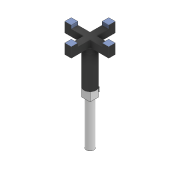
# Autodesk Inventor part: stand
Saved by Autodesk Inventor 2021 (Build 250183000, 183)
## iProperties
Created: 2021-06-25
Part Number: stand
Material: Generic
Document SubType Name: Modeling
Designer: user
Density: 1 g/cm^3
Appearance: Default
Author: user
Autodesk Inventor part; units mm, degrees
ref_plane "YZ Plane" through (0, 0, 0) normal (1, 0, 0) x (0, 1, 0)
ref_plane "XZ Plane" through (0, 0, 0) normal (0, 1, 0) x (-1, 0, 0)
ref_plane "XY Plane" through (0, 0, 0) normal (0, 0, 1) x (1, 0, 0)
sketch "Sketch1" plane through (0, 0, 0) normal (0, 1, 0) x (-1, 0, 0)
  line L0 (-127, 19.05) -> (-127, -19.05)
  line L1 (127, -19.05) -> (127, 19.05)
  line L2 (0, -127) -> (19.05, -127)
  line L3 (19.05, -127) -> (19.05, -19.05)
  line L4 (19.05, 0) -> (0, 0)
  line L5 (0, -127) -> (-19.05, -127)
  line L6 (-19.05, -127) -> (-19.05, -19.05)
  line L7 (-19.05, 0) -> (0, 0)
  line L8 (0, 0) -> (0, -127)
  line L9 (19.05, 0) -> (0, 0)
  line L10 (-19.05, 0) -> (-19.05, 127)
  line L11 (-19.05, 127) -> (19.05, 127)
  line L12 (19.05, 127) -> (19.05, 19.05)
  line L13 (-127, -19.05) -> (-19.05, -19.05)
  line L14 (19.05, -19.05) -> (127, -19.05)
  line L15 (127, 19.05) -> (19.05, 19.05)
  line L16 (-19.05, 19.05) -> (-127, 19.05)
  point P0 (127, 0)
  point P1 (-127, 0)
  point P2 (0, 19.05)
  point P3 (0, -19.05)
  dimension "d7" = 127
  dimension "d8" = 19.05
  dimension "d9" = 127
  constraints: 34 end point, 10 parallel, 5 horizontal, 5 perpendicular, 2 point on line, 1 coincident
  measures "d7" distance of L4.start L2.end
  measures "d8" distance of L4.end L7.start
  measures "d9" distance of L10.start L10.end
extrude "Extrusion1" add sketch "Sketch1" along normal blind 38.1
sketch "Sketch2" plane through (0, 38.1, 0) normal (0, 1, 0) x (1, 0, 0)
  line L0 (-19.05, -127) -> (19.05, -127) projected
  line L1 (-19.05, -127) -> (19.05, -127)
  line L2 (19.05, -127) -> (19.05, -88.9)
  line L3 (19.05, -88.9) -> (-19.05, -88.9)
  line L4 (-19.05, -88.9) -> (-19.05, -127)
  line L5 (-19.05, 127) -> (-19.05, 19.05) projected
  line L6 (19.05, 19.05) -> (19.05, 127) projected
  line L7 (-19.05, 127) -> (19.05, 127)
  line L8 (19.05, 127) -> (19.05, 88.9)
  line L9 (19.05, 88.9) -> (-19.05, 88.9)
  line L10 (-19.05, 88.9) -> (-19.05, 127)
  line L11 (-127, -19.05) -> (-19.05, -19.05) projected
  line L12 (-19.05, 19.05) -> (-127, 19.05) projected
  line L13 (-127, -19.05) -> (-88.9, -19.05)
  line L14 (-88.9, -19.05) -> (-88.9, 19.05)
  line L15 (-88.9, 19.05) -> (-127, 19.05)
  line L16 (-127, 19.05) -> (-127, -19.05)
  line L17 (127, -19.05) -> (127, 19.05) projected
  line L18 (127, 19.05) -> (19.05, 19.05) projected
  line L19 (127, -19.05) -> (88.9, -19.05)
  line L20 (88.9, -19.05) -> (88.9, 19.05)
  line L21 (88.9, 19.05) -> (127, 19.05)
  line L22 (127, 19.05) -> (127, -19.05)
  point P0 (0, 0)
  point P1 (-19.05, 88.9)
  dimension "d12" = 38.1
  dimension "d13" = 38.1
  dimension "d14" = 38.1
  dimension "d15" = 38.1
  dimension "d16" = 38.1
  constraints: 32 end point, 8 parallel, 4 horizontal, 4 perpendicular, 3 point on line
  measures "d12" distance of L3.end L2.end
  measures "d13" distance of L2.end L1.end
  measures "d14" distance of L7.end L8.end
  measures "d15" distance of L15.end L14.end
  measures "d16" distance of L20.end L21.end
extrude "Extrusion2" add sketch "Sketch2" along normal blind 19.05
sketch "Sketch3" plane through (0, 0, 0) normal (0, -1, 0) x (1, 0, 0)
  circle A0 centre (0, 0) radius 38.1
  dimension "d19" = 76.2
  constraints: 1 centre point, 1 coincident
  measures "d19" diameter of A0
extrude "Extrusion3" add sketch "Sketch3" along normal blind 25.4
sketch "Sketch4" plane through (0, -25.4, 0) normal (0, -1, 0) x (1, 0, 0)
  circle A0 centre (0, 0) radius 34.925
  dimension "d22" = 69.85
  constraints: 1 centre point, 1 coincident
  measures "d22" diameter of A0
extrude "Extrusion4" add sketch "Sketch4" along normal blind 190.5
sketch "Sketch5" plane through (0, -215.9, 0) normal (0, -1, 0) x (1, 0, 0)
  circle A0 centre (0, 0) radius 34.925 projected
  line L0 (24.9762, 24.412) -> (-24.9888, 24.412)
  line L1 (-24.9888, 24.412) -> (-24.9888, -24.3991)
  line L2 (-24.9888, -24.3991) -> (24.9762, -24.3991)
  line L3 (24.9762, -24.3991) -> (24.9762, 24.412)
  point P0 (-24.9762, 24.412)
  point P1 (-24.9888, 24.3991)
  constraints: 8 end point, 2 parallel, 2 point on circle, 1 horizontal, 1 perpendicular
extrude "Extrusion5" add sketch "Sketch5" along normal blind 50.8 contours L3 L2 L1 A0 L0
sketch "Sketch6" plane through (24.9762, -215.9, -24.3991) normal (0, 0, -1) x (-1, 0, 0)
  line L0 (11.8903, -39.6018) -> (38.7164, -39.6018)
  line L1 (38.7164, -39.6018) -> (38.7164, -13.4301)
  line L2 (38.7164, -13.4301) -> (11.8903, -13.4301)
  line L3 (11.8903, -13.4301) -> (11.8903, -39.6018)
  point P0 (24.9762, 215.9)
  constraints: 8 end point, 2 parallel, 1 horizontal, 1 perpendicular
extrude "Extrusion6" add sketch "Sketch6" along normal blind 19.05
fillet "Fillet1" radius 3.175 7 edges at (-0.3271, -255.5018, -43.4491) (13.0859, -255.5018, -33.9241) (13.0859, -242.416, -43.4491) (13.0859, -229.3301, -33.9241) (-0.3271, -229.3301, -43.4491) (-13.7402, -229.3301, -33.9241) (-13.7402, -242.416, -43.4491)
fillet "Fillet2" radius 3.175 2 edges at (-12.8102, -254.5719, -42.5191) (-13.7402, -255.5018, -32.3366)
sketch "Sketch7" plane through (0, -266.7, 0) normal (0, -1, 0) x (1, 0, 0)
  circle A0 centre (0, 0) radius 22.225
  dimension "d31" = 44.45
  constraints: 1 centre point, 1 coincident
  measures "d31" diameter of A0
extrude "Extrusion7" add sketch "Sketch7" along normal blind 254
sketch "Sketch8" plane through (0, -520.7, 0) normal (0, -1, 0) x (1, 0, 0)
  point P0 (0, 0)
body "Solid1"
